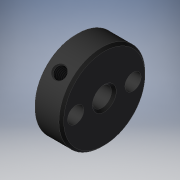
# Autodesk Inventor part: SC  0406CP2-part
Saved by Autodesk Inventor 2019 (Build 230136000, 136)
## iProperties
Created: 2022-12-12
Part Number: SC  0406CP2-part
Material: Generic
Catalog Web Link: www.cadenas.de
Description: Standard Set Collars-2 holes For fixation type-part-Standard Set Collars-2 holes For fixation type-part
Vendor: IWATA
Document SubType Name: Modeling
Designer: psAdmin
Manufacturer: IWATA
Mass: 1.29123 g
Surface Area: 9.94292 cm^2
Volume: 1.29123 cm^3
Density: 1 g/cm^3
Appearance: PSOLRGB-175-175-175
Category: PARTsolutions
Company: IWATA
Title: SC  0406CP2-part
Author: Cadenas PARTsolutions
Comments: Standard Set Collars-2 holes For fixation type-part
PSOL_IDENT_0: {$CADENAS_DATA/23d-libs/iwata/standard_set_collars/with_hole_type/2_holes/parts/ssetc_2hfft_p.prj},2
PSOL_IDENT_1: 17 {VTYP=3D},{NB=SC  0406CP2-part},{LINA=SC  0406CP2-part},{NN=Standard Set Collars-2 holes For fixa
PSOL_IDENT_2: tion type-part},{DATE=13.01.2022 05:15:09},{GEOMDATE=03.11.2008 00:00:00},{VERSION=},{LINEID=30},{WB
PSOL_IDENT_3: VAR=},{WBNUMERIC=}  {NB=SC  0406CP2-part},{LINA=SC  0406CP2-part},{KT=DUMMY},{MAT=Steel,Black},{B=4}
PSOL_IDENT_4: ,{L=6},{D=18},{S=3.4},{PCD=12},{M=M3 x 3},{ORDERNUMBER=SC  0406CP2},{SMX=C},{C=0.5},{NDM=3},{KDM=2.4
PSOL_IDENT_5: 59},{H=3},{NRH=1},{PPATH=ssetc_2hfft_asmtpl.prj}
NB: SC  0406CP2-part
NN: Standard Set Collars-2 holes For fixation type-part
NT: Standard Set Collars-2 holes For fixation type-part
NBSYN: $ORDERNUMBER.-part
LINA: SC  0406CP2-part
CATALOG: IWATA MFG. CO., LTD
MAT: Steel,Black
B: 4
L: 6
D: 18
S: 3.4
PCD: 12
SMX: C
C: 0.5
NDM: 3
KDM: 2.459
H: 3
NRH: 1
PPATH: ssetc_2hfft_asmtpl.prj
SUPPLIER: IWATA
ARTICLENO: SC  0406CP2-part
BOMINFO: SC  0406CP2-part
CREATOR: CADENAS GmbH
Autodesk Inventor part; units mm, degrees
sketch "Sketch_1" plane through (0, 0, 0) normal (0, 0, 1) x (1, 0, 0)
  line L0 (6, 0) -> (0, 0)
  line L1 (0, 2.5) -> (0.5, 2)
  line L2 (0.5, 2) -> (5.5, 2)
  line L3 (5.5, 2) -> (6, 2.5)
  line L4 (6, 2.5) -> (6, 8.5)
  line L5 (6, 8.5) -> (5.5, 9)
  line L6 (5.5, 9) -> (0.5, 9)
  line L7 (0.5, 9) -> (0, 8.5)
  line L8 (0, 8.5) -> (0, 2.5)
  constraints: 18 end point
revolve "Revolution1" add sketch "Sketch_1" angle 360 about axis through (6, 0, 0) along (1, 0, 0)
sketch "Sketch_4" plane through (3, 0, 0) normal (1, 0, 0) x (0, 0, -1)
  line L0 (-0.7071, 0.7071) -> (-6.364, 6.364)
  line L1 (-6.364, 6.364) -> (-5.3033, 7.4246)
  line L2 (-5.3033, 7.4246) -> (-5.3033, 7.0421)
  line L3 (-5.3033, 7.0421) -> (0.1623, 1.5765)
  line L4 (0.1623, 1.5765) -> (-0.7071, 0.7071)
  line L5 (-0.7071, 0.7071) -> (-6.364, 6.364)
  constraints: 12 end point
revolve "Revolution2" cut sketch "Sketch_4" angle 360 about axis through (3, 0.7071, 0.7071) along (0, -0.7071068, -0.7071068)
thread "Thread1" size "M3x0.5" class "6H" standard "ISO Metric profile" length 6.7295
sketch "Sketch_2" plane through (3, 0, 0) normal (1, 0, 0) x (0, 0, -1)
  circle A0 centre (6, 0) radius 1.7
  constraints: 1 centre point
extrude "Extrusion1" cut sketch "Sketch_2" along normal mid plane 6
sketch "Sketch_6" plane through (3, 0, 0) normal (1, 0, 0) x (0, 0, -1)
  circle A0 centre (-6, 0) radius 1.7
  constraints: 1 centre point
extrude "Extrusion2" cut sketch "Sketch_6" along normal mid plane 6
ref_plane "part_XY" through (0, 0, 0) normal (-1, 0, 0) x (0, 0, -1)
ref_plane "part_YZ" through (0, 0, 0) normal (0, 0, -1) x (0, -1, 0)
ref_plane "part_ZX" through (0, 0, 0) normal (0, -1, 0) x (-1, 0, 0)
body "Solid1"
